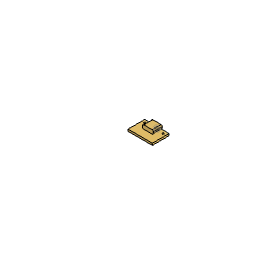
CronusPlywood (Autodesk Fusion 360 archive; units mm, degrees)
design "PwrBoard"
Autodesk Fusion 360 part; units mm, degrees
sketch "Sketch1" plane through (0, 0, 6) normal (0, 0, 1) x (-1, 0, 0)
  line L0 (-57, -24.5) -> (-77.4, -24.5)
  line L1 (-77.4, -24.5) -> (-77.4, -38.5)
  line L2 (-77.4, -38.5) -> (-57, -38.5)
  line L3 (-57, -38.5) -> (-57, -24.5)
  line L4 (-77.4, -24.5) -> (-57, -24.5)
  line L5 (-57, -24.5) -> (-57, -38.5)
  line L6 (-57, -38.5) -> (-77.4, -38.5)
  line L7 (-77.4, -38.5) -> (-77.4, -24.5)
  line L8 (-77.4, -38.5) -> (-74.8997, -35.9997) construction
  line L9 (-77.4, -38.5) -> (-73.764, -38.5) construction
  line L10 (-57, -38.5) -> (-59.5003, -35.9997) construction
  line L11 (-57, -38.5) -> (-60.436, -38.5) construction
  circle A0 centre (-74.8997, -35.9997) radius 0.75
  circle A1 centre (-59.5003, -35.9997) radius 0.75
  dimension "d144" = 3.536
  dimension "d145" = 45
  dimension "d146" = 45
  dimension "d147" = 3.536
  dimension "d148" = 1.5
  dimension "d149" = 1.5
  constraint horizontal L4
  constraint vertical L5
  constraint horizontal L6
  constraint vertical L7
  constraint coincident L2.end L3.start
  constraint coincident L0.end L1.start
  constraint horizontal L9
  constraint coincident L1.end L2.start
  constraint horizontal L11
  constraint coincident L8.end A0.centre
  constraint coincident L10.end A1.centre
  measures "d144" distance of L1.end L8.end
  measures "d145" angle of L8 L9
  measures "d146" angle of L10 L11
  measures "d147" distance of L2.end L10.end
  measures "d148" diameter of A0
  measures "d149" diameter of A1
extrude "Extrude1" add sketch "Sketch1" along normal blind 1.6 makes body 1
sketch "Sketch2" plane through (0, 0, 7.6) normal (0, 0, 1) x (-1, 0, 0)
  circle A0 centre (-59.5003, -35.9997) radius 0.75
  circle A1 centre (-74.8997, -35.9997) radius 0.75
  line L0 (-77.4, -38.5) -> (-57, -38.5)
  line L1 (-57, -38.5) -> (-57, -24.5)
  line L2 (-57, -24.5) -> (-77.4, -24.5)
  line L3 (-77.4, -24.5) -> (-77.4, -38.5)
  line L4 (-67.2, -38.5) -> (-71.7, -38.5) construction
  line L5 (-67.2, -38.5) -> (-67.2, -31) construction
  line L6 (-67.2, -31) -> (-62.7, -31) construction
  line L7 (-71.7, -38.5) -> (-62.7, -38.5)
  line L8 (-62.7, -38.5) -> (-62.7, -31)
  line L9 (-62.7, -31) -> (-71.7, -31)
  line L10 (-71.7, -31) -> (-71.7, -38.5)
  dimension "d152" = 4.5
  dimension "d153" = 7.5
  dimension "d154" = 4.5
  constraint midpoint L0 L4.start
  constraint horizontal L4
  constraint vertical L5
  constraint horizontal L6
  constraint horizontal L7
  constraint vertical L8
  constraint horizontal L9
  constraint vertical L10
  measures "d152" distance of L4.start L4.end
  measures "d153" distance of L4.start L5.end
  measures "d154" distance of L5.end L6.end
extrude "Extrude2" add sketch "Sketch2" along normal blind 3.2 separate body contours L0 L7 L8 L9 L10 makes body 2
fillet "Fillet1" radius 1 4 edges at (71.7, 34.75, 10.8) (71.7, 34.75, 7.6) (62.7, 34.75, 7.6) (62.7, 34.75, 10.8) on bodies 2
sketch "Sketch3" plane through (0, 38.5, 0) normal (0, 1, 0) x (-1, 0, 0)
  line L0 (-77.4, 6) -> (-57, 6)
  line L1 (-57, 6) -> (-57, 7.6)
  line L2 (-57, 7.6) -> (-77.4, 7.6)
  line L3 (-77.4, 7.6) -> (-77.4, 6)
  point P0 (-67.2, 6)
  constraint midpoint L0 P0
equation "d150 = pwrBoardThick"
equation "pwrBoardThick = 1.6 mm"

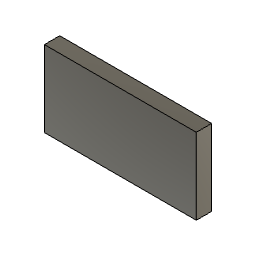
design "Display"
Autodesk Fusion 360 part; units mm, degrees
sketch "Sketch1" plane through (0, 2.4, 0) normal (0, -1, 0) x (-1, 0, 0)
  line L0 (-131.4, -67.6) -> (-3, -67.6) construction
  line L1 (-131.4, -3) -> (-131.4, -67.6) construction
  line L2 (-3, -67.6) -> (-3, -3) construction
  line L3 (-3, -3) -> (-131.4, -3) construction
  line L4 (-131.2, -3.2) -> (-131.2, -67.4)
  line L5 (-131.2, -67.4) -> (-3.2, -67.4)
  line L6 (-3.2, -67.4) -> (-3.2, -3.2)
  line L7 (-3.2, -3.2) -> (-131.2, -3.2)
extrude "Extrude1" add sketch "Sketch1" against normal blind 12.9
sketch "Sketch2" plane through (0, 15.3, 0) normal (0, 1, 0) x (-1, 0, 0)
  line L0 (-131.2, 67.4) -> (-131.2, 61.4) construction
  line L1 (-131.2, 61.4) -> (-3.2, 61.4) construction
  line L2 (-131.2, 61.4) -> (-128.2, 61.4) construction
  circle A0 centre (-128.2, 61.4) radius 1.65
  circle A1 centre (-96.2, 61.4) radius 1.65
  circle A2 centre (-64.2, 61.4) radius 1.65
  circle A3 centre (-32.2, 61.4) radius 1.65
  line L3 (-128.2, 61.4) -> (-102.2, 61.4) construction
  circle A4 centre (-102.2, 61.4) radius 1.65
  circle A5 centre (-70.2, 61.4) radius 1.65
  circle A6 centre (-38.2, 61.4) radius 1.65
  circle A7 centre (-6.2, 61.4) radius 1.65
  circle A8 centre (-128.2, 41.4) radius 1.65
  circle A9 centre (-96.2, 41.4) radius 1.65
  circle A10 centre (-64.2, 41.4) radius 1.65
  circle A11 centre (-32.2, 41.4) radius 1.65
  circle A12 centre (-102.2, 41.4) radius 1.65
  circle A13 centre (-70.2, 41.4) radius 1.65
  circle A14 centre (-38.2, 41.4) radius 1.65
  circle A15 centre (-6.2, 41.4) radius 1.65
  line L4 (-131.2, 35.3) -> (-3.2, 35.3) construction
  circle A16 centre (-128.2, 9.2) radius 1.65
  circle A17 centre (-128.2, 29.2) radius 1.65
  circle A18 centre (-102.2, 29.2) radius 1.65
  circle A19 centre (-102.2, 9.2) radius 1.65
  circle A20 centre (-96.2, 9.2) radius 1.65
  circle A21 centre (-96.2, 29.2) radius 1.65
  circle A22 centre (-70.2, 29.2) radius 1.65
  circle A23 centre (-70.2, 9.2) radius 1.65
  circle A24 centre (-64.2, 9.2) radius 1.65
  circle A25 centre (-64.2, 29.2) radius 1.65
  circle A26 centre (-38.2, 9.2) radius 1.65
  circle A27 centre (-32.2, 9.2) radius 1.65
  circle A28 centre (-38.2, 29.2) radius 1.65
  circle A29 centre (-32.2, 29.2) radius 1.65
  circle A30 centre (-6.2, 9.2) radius 1.65
  circle A31 centre (-6.2, 29.2) radius 1.65
  line L5 (-131.2, 3.2) -> (-3.2, 3.2)
  line L6 (-3.2, 3.2) -> (-3.2, 67.4)
  line L7 (-3.2, 67.4) -> (-131.2, 67.4)
  line L8 (-131.2, 67.4) -> (-131.2, 3.2)
  dimension "d20" = 6
  dimension "d21" = 3
  dimension "d22" = 3.3
  dimension "d25" = 32
  dimension "d26" = -20
  dimension "d27" = 26
  dimension "d28" = 3.3
  dimension "d31" = 32
  dimension "d32" = -20
  constraint perpendicular L0 L2
  constraint coincident L2.end A0.centre
  constraint parallel L1 L3
  constraint coincident L3.end A4.centre
  constraint symmetric A0 L4 A16
  constraint symmetric A1 L4 A20
  constraint symmetric A2 L4 A24
  constraint symmetric A3 L4 A27
  constraint symmetric A4 L4 A19
  constraint symmetric A5 L4 A23
  constraint symmetric A6 L4 A26
  constraint symmetric A7 L4 A30
  constraint symmetric A8 L4 A17
  constraint symmetric A9 L4 A21
  constraint symmetric A10 L4 A25
  constraint symmetric A11 L4 A29
  constraint symmetric A12 L4 A18
  constraint symmetric A13 L4 A22
  constraint symmetric A14 L4 A28
  constraint symmetric A15 L4 A31
  constraint coincident L1.end L6
  constraint coincident L0.end L8
  constraint coincident L0.start L7.end
  constraint midpoint L4.start L8
  constraint midpoint L4.end L6
  measures "d20" distance of L0.end L0.start
  measures "d21" distance of L0.end L2.end
  measures "d22" diameter of A0
  measures "d27" distance of L2.end L3.end
  measures "d28" diameter of A4
extrude "Extrude2" cut sketch "Sketch2" against normal blind 2 contours A0 | A1 | A2 | A3 | A4 | A5 | A6 | A7 | A8 | A9 | A10 | A11 | A12 | A13 | A14 | A15 | A16 | A17 | A18 | A19 | A20 | A21 | A22 | A23 | A24 | A25 | A26 | A27 | A28 | A29 | A30 | A31
equation "d18 = -dispThick"
equation "d51 = -tolerance"
equation "dispThick = 12.9 mm"
equation "tolerance = 0.2 mm"

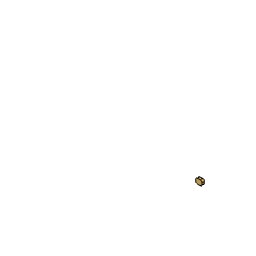
design "LightSensor"
Autodesk Fusion 360 part; units mm, degrees
sketch "Sketch1" plane through (0, 40.3, 0) normal (0, 1, 0) x (-1, 0, 0)
  line L0 (-131.4, 3) -> (-131.4, 67.6)
  line L1 (-131.4, 67.6) -> (-3, 67.6) construction
  line L2 (-3, 67.6) -> (-3, 3)
  line L3 (-3, 3) -> (-131.4, 3)
  line L4 (0, 70.6) -> (-134.4, 70.6)
  line L5 (-134.4, 70.6) -> (-134.4, 0)
  line L6 (-134.4, 0) -> (0, 0)
  line L7 (0, 0) -> (0, 70.6)
  line L8 (-131.4, 67.6) -> (-3, 67.6)
  line L9 (-69.675, 67.6) -> (-64.725, 67.6) construction
  line L10 (-64.725, 67.6) -> (-64.725, 60.6) construction
  line L11 (-64.725, 60.6) -> (-69.675, 60.6) construction
  line L12 (-69.675, 60.6) -> (-69.675, 67.6) construction
  line L13 (-68.425, 60.6) -> (-65.975, 60.6)
  line L14 (-64.725, 61.85) -> (-64.725, 63.35)
  line L15 (-65.975, 64.6) -> (-68.425, 64.6)
  line L16 (-69.675, 63.35) -> (-69.675, 61.85)
  arc A0 (-68.425, 64.6) -> (-69.675, 63.35) centre (-68.425, 63.35) ccw
  arc A1 (-69.675, 61.85) -> (-68.425, 60.6) centre (-68.425, 61.85) ccw
  arc A2 (-65.975, 60.6) -> (-64.725, 61.85) centre (-65.975, 61.85) ccw
  arc A3 (-64.725, 63.35) -> (-65.975, 64.6) centre (-65.975, 63.35) ccw
  point P0 (-69.675, 64.6)
  dimension "d159" = 4.95
  dimension "d160" = 7
  dimension "d161" = 4
  dimension "d162" = 1.25
  dimension "d163" = 1.25
  dimension "d164" = 1.25
  dimension "d165" = 1.25
  constraint horizontal L9
  constraint vertical L10
  constraint horizontal L11
  constraint vertical L12
  constraint coincident L8 L9.start
  constraint midpoint L8 L9
  constraint horizontal L13
  constraint vertical L14
  constraint horizontal L15
  constraint vertical L16
  constraint coincident P0 L15
  constraint coincident P0 L16
  constraint tangent L15 A0
  constraint tangent L16 A0
  constraint coincident L11.end L13
  constraint coincident L11.end L16
  constraint tangent L13 A1
  constraint tangent L16 A1
  constraint tangent L13 A2
  constraint tangent L14 A2
  constraint tangent L15 A3
  constraint tangent L14 A3
  measures "d159" distance of L9.start L9.end
  measures "d160" distance of L9.start L11.end
  measures "d161" distance of L11.end P0
  measures "d162" radius of A0
  measures "d163" radius of A1
  measures "d164" radius of A2
  measures "d165" radius of A3
extrude "Extrude1" add sketch "Sketch1" against normal blind 1.9 contours L13 L14 L15 L16 A0 A1 A2 A3
equation "d160 = 4 mm + wallThick"
equation "wallThick = 3 mm"
